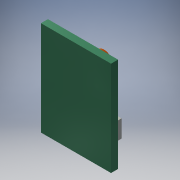
# Autodesk Inventor part: CdS모듈
Saved by Autodesk Inventor 2017 (Build 210142000, 142)
## iProperties
Part Number: CdS모듈
Material: 일반
Document SubType Name: Modeling
Designer: minom
Density: 1 g/cm^3
Appearance: 기본값
Author: minom
Autodesk Inventor part; units mm, degrees
ref_plane "YZ Plane" through (0, 0, 0) normal (1, 0, 0) x (0, 1, 0)
ref_plane "XZ Plane" through (0, 0, 0) normal (0, 1, 0) x (-1, 0, 0)
ref_plane "XY Plane" through (0, 0, 0) normal (0, 0, 1) x (1, 0, 0)
sketch "스케치1" plane through (0, 0, 0) normal (0, 1, 0) x (-1, 0, 0)
  line L0 (0, 0) -> (-20, 0)
  line L1 (-20, 0) -> (-20, -27)
  line L2 (-20, -27) -> (0, -27)
  line L3 (0, -27) -> (0, 0)
  dimension "d0" = 20
  dimension "d1" = 27
  constraints: 8 end point, 2 parallel, 1 horizontal, 1 perpendicular
  measures "d0" distance of L2.end L1.end
  measures "d1" distance of L1.end L0.end
extrude "돌출1" add sketch "스케치1" along normal blind 2
sketch "스케치2" plane through (0, 2, 0) normal (0, 1, 0) x (1, 0, 0)
  line L0 (0, 0) -> (20, 0) projected
  line L1 (20, 0) -> (20, 27) projected
  line L2 (20, 27) -> (0, 27) projected
  line L3 (0, 27) -> (0, 0) projected
  line L4 (5, 20) -> (15, 20)
  line L5 (15, 20) -> (15, 25)
  line L6 (15, 25) -> (5, 25)
  line L7 (5, 25) -> (5, 20)
  dimension "d4" = 5
  dimension "d5" = 2
  dimension "d6" = 5
  dimension "d7" = 10
  constraints: 8 end point, 2 parallel, 1 horizontal, 1 perpendicular
  measures "d4" distance between parallel lines of L7 L3
  measures "d5" distance between parallel lines of L6 L2
  measures "d6" distance between parallel lines of L4 L6
  measures "d7" distance between parallel lines of L5 L7
extrude "돌출2" add sketch "스케치2" along normal blind 6 contours L7 L6 L5 L4
sketch "스케치3" plane through (0, 2, 0) normal (0, 1, 0) x (1, 0, 0)
  line L0 (5, 20) -> (5, 25) projected
  line L1 (5, 25) -> (15, 25) projected
  line L2 (15, 25) -> (15, 20) projected
  line L3 (15, 20) -> (5, 20) projected
  line L4 (0, 0) -> (20, 0) projected
  line L5 (20, 0) -> (20, 27) projected
  line L6 (20, 27) -> (0, 27) projected
  line L7 (0, 27) -> (0, 0) projected
  circle A0 centre (10, 8) radius 2.5
  dimension "d10" = 5
  dimension "d11" = 8
  constraints: 1 centre point
  measures "d10" diameter of A0
  measures "d11" distance from line of L4 A0.centre
extrude "돌출3" add sketch "스케치3" along normal blind 6 contours A0
sketch "스케치4" plane through (0, 2, 0) normal (0, 1, 0) x (1, 0, 0)
  circle A0 centre (10, 8) radius 2.5 projected
  line L0 (5, 20) -> (5, 25) projected
  line L1 (5, 25) -> (15, 25) projected
  line L2 (15, 25) -> (15, 20) projected
  line L3 (15, 20) -> (5, 20) projected
  line L4 (0, 0) -> (20, 0) projected
  line L5 (20, 0) -> (20, 27) projected
  line L6 (20, 27) -> (0, 27) projected
  line L7 (0, 27) -> (0, 0) projected
  circle A1 centre (5, 16) radius 1.5
  circle A2 centre (15, 16) radius 1.5
  dimension "d14" = 3
  dimension "d15" = 3
  dimension "d16" = 5
  dimension "d17" = 11
  dimension "d18" = 11
  dimension "d19" = 5
  constraints: 2 centre point
  measures "d14" diameter of A1
  measures "d15" diameter of A2
  measures "d16" distance from line of A1.centre L7
  measures "d17" distance from line of L6 A1.centre
  measures "d18" distance from line of L6 A2.centre
  measures "d19" distance from line of L5 A2.centre
extrude "돌출4" cut sketch "스케치4" against normal blind 6 contours A1 | A2
